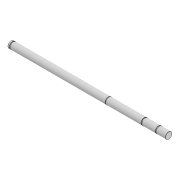
# Autodesk Inventor part: Long shaft2
Saved by Autodesk Inventor 2021 (Build 250183000, 183)
## iProperties
Created: 2020-10-30
Part Number: Long shaft2
Material: Generic
Document SubType Name: Modeling
Designer: Alfred Brauner
Density: 1 g/cm^3
Appearance: Default
Author: Alfred Brauner
Autodesk Inventor part; units mm, degrees
ref_plane "YZ Plane" through (0, 0, 0) normal (1, 0, 0) x (0, 1, 0)
ref_plane "XZ Plane" through (0, 0, 0) normal (0, 1, 0) x (-1, 0, 0)
ref_plane "XY Plane" through (0, 0, 0) normal (0, 0, 1) x (1, 0, 0)
sketch "Sketch1" plane through (0, 0, 0) normal (0, 0, 1) x (1, 0, 0)
  line L0 (0, 0) -> (0, 5)
  line L1 (0, 5) -> (-14.25, 5)
  line L2 (-14.25, 5) -> (-14.25, 4.5)
  line L3 (-14.25, 4.5) -> (-15.35, 4.5)
  line L4 (-15.35, 4.5) -> (-15.35, 5)
  line L5 (-15.35, 5) -> (-35.85, 5)
  line L6 (-35.85, 5) -> (-35.85, 4.5)
  line L7 (-35.85, 4.5) -> (-36.95, 4.5)
  line L8 (-36.95, 4.5) -> (-36.95, 5)
  line L9 (-235.2, 0) -> (0, 0)
  line L10 (-36.95, 5) -> (-90.4, 5)
  line L11 (-90.4, 5) -> (-90.4, 4.5)
  line L12 (-90.4, 4.5) -> (-91.5, 4.5)
  line L13 (-91.5, 4.5) -> (-91.5, 5)
  line L14 (-91.5, 5) -> (-235.2, 5)
  line L15 (-235.2, 5) -> (-235.2, 4.5)
  line L16 (-235.2, 4.5) -> (-236.3, 4.5)
  line L17 (-236.3, 4.5) -> (-236.3, 5)
  line L18 (-236.3, 5) -> (-238.3, 5)
  line L19 (-238.3, 5) -> (-238.3, 0)
  line L20 (-238.3, 0) -> (-235.2, 0)
  dimension "d0" = 5
  dimension "d1" = 0.5
  dimension "d2" = 1.1
  dimension "d3" = 1.1
  dimension "d4" = 15.35
  dimension "d6" = 35.85
  dimension "d11" = 1.1
  dimension "d12" = 91.5
  dimension "d13" = 1.1
  dimension "d14" = 2
  dimension "d15" = 238.3
  constraints: 42 end point, 12 perpendicular, 7 point on line, 3 horizontal, 1 collinear, 1 parallel, 1 vertical
  measures "d0" distance of L0.start L0.end
  measures "d1" distance of L1.end L2.end
  measures "d2" distance of L2.end L3.end
  measures "d3" distance of L6.end L7.end
  measures "d4" distance between parallel lines of L4 L0
  measures "d6" distance between parallel lines of L6 L0
  measures "d11" distance of L11.end L12.end
  measures "d12" distance between parallel lines of L13 L0
  measures "d13" distance of L15.end L16.end
  measures "d14" distance of L17.end L18.end
  measures "d15" distance between parallel lines of L0 L19
revolve "Revolution1" add sketch "Sketch1" angle 360 about axis through (-235.2, 0, 0) along (1, 0, 0)
chamfer "Chamfer1" distance 0.2 angle 45 6 edges at (-235.2, -5, 0) (-35.85, -5, 0) (-36.95, -5, 0) (-14.25, -5, 0) (-15.35, -5, 0) (0, -5, 0)
body "Solid1"
